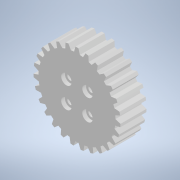
# Autodesk Inventor part: Pinion
Saved by Autodesk Inventor 2021 (Build 250183000, 183)
## iProperties
Created: 2025-04-11
Part Number: Pinion
Material: Generic
Document SubType Name: Modeling
Designer: Lukas
Density: 1 g/cm^3
Appearance: Default
Author: Lukas
Autodesk Inventor part; units mm, degrees
ref_plane "YZ Plane" through (0, 0, 0) normal (1, 0, 0) x (0, 1, 0)
ref_plane "XZ Plane" through (0, 0, 0) normal (0, 1, 0) x (-1, 0, 0)
ref_plane "XY Plane" through (0, 0, 0) normal (0, 0, 1) x (1, 0, 0)
sketch "Sketch1" plane through (0, 0, 0) normal (0, 0, 1) x (1, 0, 0)
  circle A0 centre (-4.25, 4.25) radius 1.15
  circle A1 centre (4.25, 4.25) radius 1.15
  circle A2 centre (4.25, -4.25) radius 1.15
  circle A3 centre (-4.25, -4.25) radius 1.15
  circle A4 centre (0, 0) radius 15.5
  line L0 (-1.1731, 15.4555) -> (-0.6, 17.5)
  line L1 (-0.6, 17.5) -> (0.6, 17.5)
  line L2 (0.6, 17.5) -> (1.1731, 15.4555)
  line L3 (-1.1731, 15.4555) -> (0, 0)
  circle A5 centre (0, 0) radius 14
  circle A6 centre (-4.25, 4.25) radius 2.1
  circle A7 centre (4.25, 4.25) radius 2.1
  circle A8 centre (4.25, -4.25) radius 2.1
  circle A9 centre (-4.25, -4.25) radius 2.1
  point P0 (0, 17.5)
  dimension "d0" = 8.5
  dimension "d1" = 4.25
  dimension "d2" = 8.5
  dimension "d3" = 4.25
  dimension "d4" = 2.3
  dimension "d6" = 1.2
  dimension "d7" = 20
  dimension "d8" = 2
  dimension "d9" = 1.5
  dimension "d10" = 4.2
  dimension "d20" = 28
  constraints: 10 centre point, 8 end point, 6 coincident, 6 equal radius, 3 vertical alignment, 2 horizontal alignment, 2 point on circle, 1 equal length, 1 horizontal, 1 midpoint
  measures "d0" distance of A1.centre A0.centre
  measures "d1" horizontal distance of A0.centre point (0, 0)
  measures "d2" distance of A3.centre A0.centre
  measures "d3" horizontal distance of A0.centre point (0, 0)
  measures "d4" diameter of A0
  measures "d6" distance of L0.end L1.end
  measures "d7" angle of L0 L3
  measures "d8" distance edge to line of A4 L1
  measures "d9" radial gap between concentric circles of A4 A5
  measures "d10" diameter of A6
  measures "d20" diameter of A5
extrude "Extrusion1" add sketch "Sketch1" along normal blind 1 contours A5 | A6 | A7 | A8 | A9
extrude "Extrusion2" add sketch "Sketch1" along normal blind 2.5 contours A5
extrude "Extrusion3" add sketch "Sketch1" along normal blind 2.5 and the other way blind 8 contours A4 | A4 L0 L1 L2
pattern_circular "Circular Pattern1" count 27 over 360 about axis through (0, 0, -10) along (0, 0, 1) of "Extrusion3"
equation "\"d1\" = 0.5 * d0"
equation "\"d2\" = d0"
equation "\"d3\" = 0.5 * d2"
body "Solid1"
